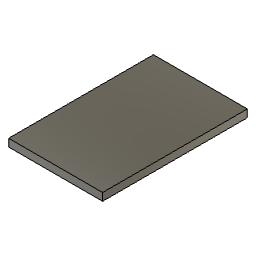
main v7 (Autodesk Fusion 360 archive; units mm, degrees)
design "中板"
Autodesk Fusion 360 part; units mm, degrees
sketch "スケッチ1" plane through (0, 0, 0) normal (0, 0, 1) x (1, 0, 0)
  line L0 (0, 0) -> (185, 0)
  line L1 (185, 0) -> (185, 285)
  line L2 (185, 285) -> (0, 285)
  line L3 (0, 285) -> (0, 0)
  dimension "d1" = 185
  dimension "d2" = 285
  constraint horizontal L0
  constraint vertical L1
  constraint horizontal L2
  constraint vertical L3
  constraint coincident L0.start L3.end
  measures "d1" distance of L1.end L2.end
  measures "d2" distance of L0.start L2.end
extrude "押し出し1" add sketch "スケッチ1" along normal blind 15

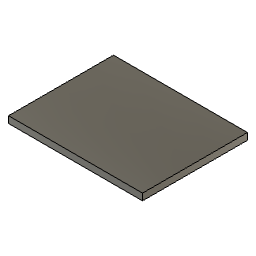
design "側板"
Autodesk Fusion 360 part; units mm, degrees
sketch "スケッチ1" plane through (0, 0, 0) normal (0, 0, 1) x (1, 0, 0)
  line L0 (0, 0) -> (300, 0)
  line L1 (300, 0) -> (300, 235)
  line L2 (300, 235) -> (0, 235)
  line L3 (0, 235) -> (0, 0)
  dimension "d1" = 300
  dimension "d2" = 235
  constraint horizontal L0
  constraint vertical L1
  constraint horizontal L2
  constraint vertical L3
  constraint coincident L0.start L3.end
  measures "d1" distance of L1.end L2.end
  measures "d2" distance of L0 L2
extrude "押し出し1" add sketch "スケッチ1" along normal blind 15

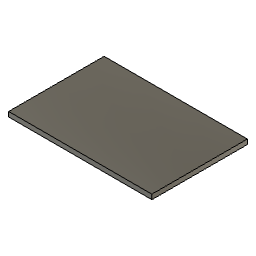
design "天板"
Autodesk Fusion 360 part; units mm, degrees
sketch "スケッチ1" plane through (0, 0, 0) normal (0, 0, 1) x (1, 0, 0)
  line L0 (0, 0) -> (450, 0)
  line L1 (450, 0) -> (450, 300)
  line L2 (450, 300) -> (0, 300)
  line L3 (0, 300) -> (0, 0)
  constraint horizontal L0
  constraint vertical L1
  constraint horizontal L2
  constraint vertical L3
  constraint coincident L0.start L3.end
extrude "押し出し1" add sketch "スケッチ1" along normal blind 15

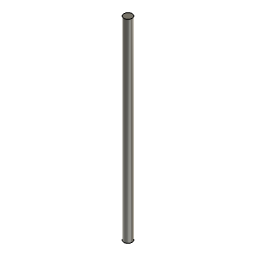
design "円柱"
Autodesk Fusion 360 part; units mm, degrees
sketch "スケッチ1" plane through (0, 0, 0) normal (0, 0, 1) x (1, 0, 0) in component "Component'"
  circle A0 centre (0, 0) radius 5
  constraint coincident A0.centre origin
extrude "押し出し1" add sketch "スケッチ1" along normal blind 235 in component "Component'"
component "Component'" placed x (1, 0, 0) y (0, 1, 0) z (0, 0, 1) at (0, 0, 0)

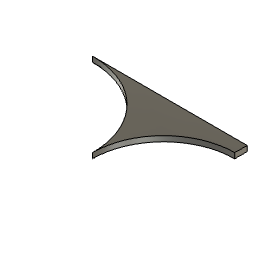
design "背面"
Autodesk Fusion 360 part; units mm, degrees
sketch "スケッチ1" plane through (0, 0, 0) normal (0, 0, 1) x (1, 0, 0)
  line L0 (0, 0) -> (435, 0)
  line L1 (435, 0) -> (435, 235)
  line L2 (435, 235) -> (0, 235)
  line L3 (0, 235) -> (0, 0)
  circle A0 centre (0, 0) radius 235
  circle A1 centre (435, 0) radius 200
  dimension "d1" = 435
  dimension "d2" = 235
  constraint horizontal L0
  constraint vertical L1
  constraint horizontal L2
  constraint vertical L3
  constraint coincident L0.start L3.end
  constraint coincident L2.end A0
  constraint coincident L0.end L1.start
  constraint tangent A0 A1
  measures "d1" distance of L1.end L2.end
  measures "d2" distance of L0.start L2.end
extrude "押し出し1" add sketch "スケッチ1" along normal blind 15 contours L1 L2 A0 A1
